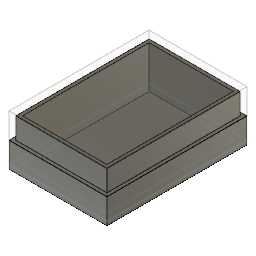
pin_box (Autodesk Fusion 360 design; units mm, degrees)
Autodesk Fusion 360 part; units mm, degrees
sketch "Sketch1" plane through (0, 0, 0) normal (0, 0, 1) x (1, 0, 0)
  line L0 (-40, 50) -> (6.4, 50)
  line L1 (6.4, 50) -> (6.4, -16.4)
  line L2 (6.4, -16.4) -> (-40, -16.4)
  line L3 (-40, -16.4) -> (-40, 50)
  line L4 (-36.8, 46.8) -> (3.2, 46.8)
  line L5 (3.2, 46.8) -> (3.2, -13.2)
  line L6 (3.2, -13.2) -> (-36.8, -13.2)
  line L7 (-36.8, -13.2) -> (-36.8, 46.8)
  dimension "d1" = 46.4
  dimension "d2" = 66.4
  dimension "d3" = 40
  dimension "d4" = 60
  dimension "d5" = 3.2
  dimension "d6" = 3.2
  constraint horizontal L0
  constraint vertical L1
  constraint horizontal L2
  constraint vertical L3
  constraint horizontal L4
  constraint vertical L5
  constraint horizontal L6
  constraint vertical L7
  measures "d1" distance of L0.start L0.end
  measures "d2" distance of L0.start L2.end
  measures "d3" distance of L4.start L4.end
  measures "d4" distance of L4.start L6.end
  measures "d5" distance of L3 L7
  measures "d6" distance of L0 L4
extrude "Extrude1" add sketch "Sketch1" against normal blind 2 contours L0 L1 L2 L3 | L4 L5 L6 L7 makes body 1
extrude "Extrude2" add sketch "Sketch1" along normal blind 10 bodies 1
sketch "Sketch2" plane through (0, 0, 10) normal (0, 0, 1) x (-1, 0, 0)
  line L0 (-3.2, 13.2) -> (36.8, 13.2)
  line L1 (36.8, 13.2) -> (36.8, -46.8)
  line L2 (36.8, -46.8) -> (-3.2, -46.8)
  line L3 (-3.2, -46.8) -> (-3.2, 13.2)
  line L4 (40, 16.4) -> (-6.4, 16.4)
  line L5 (-6.4, 16.4) -> (-6.4, -50)
  line L6 (-6.4, -50) -> (40, -50)
  line L7 (40, -50) -> (40, 16.4)
  line L8 (36.8, -46.8) -> (-3.2, -46.8)
  line L9 (-3.2, -46.8) -> (-3.2, 13.2)
  line L10 (-3.2, 13.2) -> (36.8, 13.2)
  line L11 (36.8, 13.2) -> (36.8, -46.8)
  line L12 (38.4, -48.4) -> (-4.8, -48.4)
  line L13 (-4.8, -48.4) -> (-4.8, 14.8)
  line L14 (-4.8, 14.8) -> (38.4, 14.8)
  line L15 (38.4, 14.8) -> (38.4, -48.4)
  dimension "d11" = 43.2
  dimension "d12" = 63.2
  dimension "d13" = 1.6
  dimension "d14" = 1.6
  constraint horizontal L8
  constraint vertical L9
  constraint horizontal L10
  constraint vertical L11
  constraint coincident L0.start L3.end
  constraint coincident L1.end L2.start
  constraint horizontal L12
  constraint vertical L13
  constraint horizontal L14
  constraint vertical L15
  measures "d11" distance of L12.start L12.end
  measures "d12" distance of L12.start L14.end
  measures "d13" distance of L11 L15
  measures "d14" distance of L8 L12
extrude "Extrude3" add sketch "Sketch2" along normal blind 10 contours L12 L13 L14 L15 bodies 1
sketch "Sketch3" plane through (0, 0, 20) normal (0, 0, 1) x (-1, 0, 0)
  line L0 (-3.2, 13.2) -> (36.8, 13.2)
  line L1 (36.8, 13.2) -> (36.8, -46.8)
  line L2 (36.8, -46.8) -> (-3.2, -46.8)
  line L3 (-3.2, -46.8) -> (-3.2, 13.2)
  line L4 (38.4, 14.8) -> (-4.8, 14.8)
  line L5 (-4.8, 14.8) -> (-4.8, -48.4)
  line L6 (-4.8, -48.4) -> (38.4, -48.4)
  line L7 (38.4, -48.4) -> (38.4, 14.8)
  line L8 (40, -50) -> (-6.4, -50)
  line L9 (-6.4, -50) -> (-6.4, 16.4)
  line L10 (-6.4, 16.4) -> (40, 16.4)
  line L11 (40, 16.4) -> (40, -50)
  line L12 (38.4, -48.4) -> (-4.8, -48.4)
  line L13 (-4.8, -48.4) -> (-4.8, 14.8)
  line L14 (-4.8, 14.8) -> (38.4, 14.8)
  line L15 (38.4, 14.8) -> (38.4, -48.4)
  dimension "d17" = 46.4
  dimension "d18" = 66.4
  constraint horizontal L8
  constraint vertical L9
  constraint horizontal L10
  constraint vertical L11
  constraint horizontal L12
  constraint vertical L13
  constraint horizontal L14
  constraint vertical L15
  constraint coincident L4.end L5.start
  constraint coincident L6.end L7.start
  measures "d17" distance of L8.start L8.end
  measures "d18" distance of L8.start L10.end
extrude "Extrude1'" add sketch "Sketch3" against normal blind 10 separate body contours L8 L9 L10 L11 makes body 2 in component "Component"
sketch "Sketch4" plane through (0, 0, 20) normal (0, 0, 1) x (-1, 0, 0)
  line L0 (-4.8, 14.8) -> (38.4, 14.8)
  line L1 (38.4, 14.8) -> (38.4, -48.4)
  line L2 (38.4, -48.4) -> (-4.8, -48.4)
  line L3 (-4.8, -48.4) -> (-4.8, 14.8)
  line L4 (40, 16.4) -> (-6.4, 16.4)
  line L5 (-6.4, 16.4) -> (-6.4, -50)
  line L6 (-6.4, -50) -> (40, -50)
  line L7 (40, -50) -> (40, 16.4)
  line L8 (40, -50) -> (-6.4, -50)
  line L9 (-6.4, -50) -> (-6.4, 16.4)
  line L10 (-6.4, 16.4) -> (40, 16.4)
  line L11 (40, 16.4) -> (40, -50)
  constraint horizontal L8
  constraint vertical L9
  constraint horizontal L10
  constraint vertical L11
  constraint coincident L4.end L5.start
  constraint coincident L6.end L7.start
copy_body "Body->Comp1" bodies 1 removing the originals makes body 3 in component "Component'"
sketch "Sketch5" plane through (0, 0, 20) normal (0, 0, 1) x (-1, 0, 0)
  line L0 (-4.8, 14.8) -> (38.4, 14.8)
  line L1 (38.4, 14.8) -> (38.4, -48.4)
  line L2 (38.4, -48.4) -> (-4.8, -48.4)
  line L3 (-4.8, -48.4) -> (-4.8, 14.8)
  line L4 (40, 16.4) -> (-6.4, 16.4)
  line L5 (-6.4, 16.4) -> (-6.4, -50)
  line L6 (-6.4, -50) -> (40, -50)
  line L7 (40, -50) -> (40, 16.4)
  line L8 (40, -50) -> (-6.4, -50)
  line L9 (-6.4, -50) -> (-6.4, 16.4)
  line L10 (-6.4, 16.4) -> (40, 16.4)
  line L11 (40, 16.4) -> (40, -50)
  constraint horizontal L8
  constraint vertical L9
  constraint horizontal L10
  constraint vertical L11
  constraint coincident L4.end L5.start
  constraint coincident L6.end L7.start
extrude "Extrude2'" add sketch "Sketch5" along normal blind 2 contours L0 L1 L2 L3 | L4 L5 L6 L7 L8 L9 L10 L11 bodies 2 in component "Component"
component "Component" placed x (1, 0, 0) y (0, 1, 0) z (0, 0, 1) at (0, 0, 0)
component "Component'" placed x (1, 0, 0) y (0, 1, 0) z (0, 0, 1) at (0, 0, 0)
